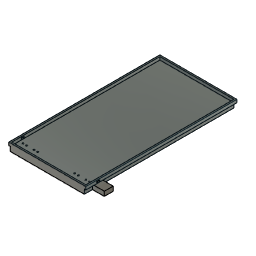
DespotovIdealisticniStoPreKampa v7 (Autodesk Fusion 360 design; units mm, degrees)
Autodesk Fusion 360 part; units mm, degrees
sketch "Sketch1" plane through (0, 0, 0) normal (0, 0, 1) x (1, 0, 0)
  line L0 (0, 0) -> (50, 0)
  line L1 (50, 0) -> (50, 100)
  line L2 (50, 100) -> (0, 100)
  line L3 (0, 100) -> (0, 0)
  constraint horizontal L0
  constraint vertical L1
  constraint horizontal L2
  constraint vertical L3
  constraint coincident L0.start L3.end
extrude "Extrude1" add sketch "Sketch1" along normal blind 3 makes body 1
sketch "Sketch2" plane through (0, 0, 3) normal (0, 0, 1) x (-1, 0, 0)
  line L0 (0, -100) -> (0, 0)
  line L1 (0, 0) -> (-50, 0)
  line L2 (-50, 0) -> (-50, -100)
  line L3 (-50, -100) -> (0, -100)
  line L4 (-50, 0) -> (0, 0)
  line L5 (0, 0) -> (0, 1)
  line L6 (0, 1) -> (-50, 1)
  line L7 (-50, 1) -> (-50, 0)
  line L8 (0, 1) -> (1, 1)
  line L9 (1, 1) -> (1, -100)
  line L10 (1, -100) -> (0, -100)
  line L11 (0, -100) -> (0, 1)
  line L12 (-50, 1) -> (-51, 1)
  line L13 (-51, 1) -> (-51, -100)
  line L14 (-51, -100) -> (-50, -100)
  line L15 (-50, -100) -> (-50, 1)
  line L16 (-51, -100) -> (1, -100)
  line L17 (1, -100) -> (1, -101)
  line L18 (1, -101) -> (-51, -101)
  line L19 (-51, -101) -> (-51, -100)
  constraint horizontal L4
  constraint vertical L5
  constraint horizontal L6
  constraint vertical L7
  constraint coincident L1.end L2.start
  constraint horizontal L8
  constraint vertical L9
  constraint horizontal L10
  constraint vertical L11
  constraint horizontal L12
  constraint vertical L13
  constraint horizontal L14
  constraint vertical L15
  constraint horizontal L16
  constraint vertical L17
  constraint horizontal L18
  constraint vertical L19
extrude "Extrude2" add sketch "Sketch2" along normal blind 2 separate body contours L3 L10 L14 L16 L17 L18 L19 | L0 L5 L8 L9 L10 L11 L16 | L1 L4 L5 L6 L7 L11 L15 | L2 L7 L12 L13 L14 L15 L16 makes body 2
sketch "Sketch3" plane through (0, 0, 3) normal (0, 0, 1) x (-1, 0, 0)
  line L0 (0, -100) -> (0, 0)
  line L1 (0, 0) -> (-50, 0)
  line L2 (-50, 0) -> (-50, -100)
  line L3 (-50, -100) -> (0, -100)
  circle A0 centre (-25, -0.9724) radius 1.0004
extrude "Extrude3" cut sketch "Sketch3" against normal blind 6 contours L1 A0 picked at (-24.8419, -0.7217) bodies 1
sketch "Sketch4" plane through (0, 0, 3) normal (0, 0, 1) x (-1, 0, 0)
  arc A0 (-25.2348, 0) -> (-24.7652, 0) centre (-25, -0.9724) ccw
  line L0 (-25.2348, 0) -> (-50, 0)
  line L1 (-50, 0) -> (-50, -100)
  line L2 (-50, -100) -> (0, -100)
  line L3 (0, -100) -> (0, 0)
  line L4 (0, 0) -> (-24.7652, 0)
  line L5 (-50, 0) -> (0, 0)
  line L6 (0, 0) -> (0, -2)
  line L7 (0, -2) -> (-50, -2)
  line L8 (-50, -2) -> (-50, 0)
  constraint horizontal L5
  constraint vertical L6
  constraint horizontal L7
  constraint vertical L8
  constraint coincident L3 L6.end
  constraint coincident L0.end L1.start
extrude "Extrude4" cut sketch "Sketch4" against normal blind 5 contours A0 L0 L1 L3 L4 L5 L6 L7 L8 bodies 1
sketch "Sketch5" plane through (0, 2, 0) normal (0, -1, 0) x (1, 0, 0)
  line L0 (0, 0) -> (50, 0)
  line L1 (50, 0) -> (50, 3)
  line L2 (50, 3) -> (0, 3)
  line L3 (0, 3) -> (0, 0)
  line L4 (23, 0) -> (0, 3)
  line L5 (0, 0) -> (0, 3)
  line L6 (0, 0) -> (23, 0)
  line L7 (27, 0) -> (50, 3)
  line L8 (50, 0) -> (50, 3)
  line L9 (50, 0) -> (27, 0)
  constraint coincident L0 L4.start
  constraint coincident L2.end L3.start
  constraint coincident L0.start L3.end
  constraint perpendicular L5 L6
  constraint coincident L0 L7.start
  constraint coincident L1.end L2.start
  constraint coincident L0.end L1.start
extrude "Extrude5" add sketch "Sketch5" along normal blind 2 contours L0 L1 L7 L8 L9 bodies 1 2
sketch "Sketch6" plane through (0, 2, 0) normal (0, -1, 0) x (1, 0, 0)
  line L0 (27, 0) -> (50, 3)
  line L1 (50, 3) -> (0, 3)
  line L2 (0, 3) -> (0, 0)
  line L3 (0, 0) -> (27, 0)
  line L4 (23, 0) -> (0, 3)
  line L5 (0, 0) -> (0, 3)
  line L6 (0, 0) -> (23, 0)
  constraint coincident L3 L4.start
  constraint coincident L1.end L2.start
  constraint coincident L2.end L3.start
  constraint perpendicular L5 L6
extrude "Extrude6" add sketch "Sketch6" along normal blind 2 separate body contours L2 L3 L4 L5 L6 makes body 3
sketch "Sketch7" plane through (0, 0, 0) normal (0, -1, 0) x (1, 0, 0)
  line L0 (0, 0) -> (23, 0)
  line L1 (23, 0) -> (0, 3)
  line L2 (0, 3) -> (0, 0)
  line L3 (0, 3) -> (50, 3)
  line L4 (50, 3) -> (50, 0)
  line L5 (50, 0) -> (0, 0)
  line L6 (0, 0) -> (0, 3)
  constraint horizontal L3
  constraint vertical L4
  constraint horizontal L5
  constraint vertical L6
  constraint coincident L1.end L2.start
extrude "Extrude7" add sketch "Sketch7" along normal blind 1 bodies 3 1
sketch "Sketch8" plane through (51, 0, 0) normal (1, 0, 0) x (0, 1, 0)
  line L0 (-1, 3) -> (101, 3)
  line L1 (101, 3) -> (101, 5)
  line L2 (101, 5) -> (-1, 5)
  line L3 (-1, 5) -> (-1, 3)
sketch "Sketch9" plane through (0, 0, 3) normal (0, 0, 1) x (-1, 0, 0)
  line L0 (0, -2) -> (-50, -2)
  line L1 (-50, -2) -> (-50, -100)
  line L2 (-50, -100) -> (0, -100)
  line L3 (0, -100) -> (0, -2)
  circle A0 centre (-47.5, -5) radius 0.5
  circle A1 centre (-45, -5) radius 0.5
  circle A2 centre (-40, -5) radius 0.5
  circle A3 centre (-37.5, -5) radius 0.5
  circle A4 centre (-2.5, -5) radius 0.5
  circle A5 centre (-5, -5) radius 0.5
  circle A6 centre (-10, -5) radius 0.5
  circle A7 centre (-12.5, -5) radius 0.5
  dimension "d15" = 1
  dimension "d16" = 1
  dimension "d17" = 1
  dimension "d18" = 1
  dimension "d19" = 1
  dimension "d20" = 1
  dimension "d21" = 1
  dimension "d22" = 1
  measures "d15" diameter of A0
  measures "d16" diameter of A1
  measures "d17" diameter of A2
  measures "d18" diameter of A3
  measures "d19" diameter of A4
  measures "d20" diameter of A5
  measures "d21" diameter of A6
  measures "d22" diameter of A7
extrude "Extrude8" cut sketch "Sketch9" against normal blind 5 contours A0 | A1 | A2 | A3 | A4 | A5 | A6 | A7 bodies 3
sketch "Sketch10" plane through (51, 0, 0) normal (1, 0, 0) x (0, 1, 0)
  circle A0 centre (8, 4) radius 0.5
  line L0 (7, 4.5) -> (6.5, 4.5)
  line L1 (6.5, 4.5) -> (6.5, 3.5)
  line L2 (6.5, 3.5) -> (7, 3.5)
  line L3 (7, 3.5) -> (7, 4.5)
  dimension "d25" = 1
  constraint horizontal L0
  constraint vertical L1
  constraint horizontal L2
  constraint vertical L3
  measures "d25" diameter of A0
extrude "Extrude9" cut sketch "Sketch10" against normal blind 500 bodies 3
sketch "Sketch11" plane through (50, 0, 0) normal (1, 0, 0) x (0, 1, 0)
  line L0 (-1, 0) -> (100, 0)
  line L1 (100, 0) -> (100, 3)
  line L2 (100, 3) -> (2, 3)
  line L3 (2, 3) -> (0, 3)
  line L4 (0, 3) -> (-1, 3)
  line L5 (-1, 3) -> (-1, 0)
sketch "Sketch12" plane through (50, 0, 0) normal (1, 0, 0) x (0, 1, 0)
  line L0 (4.5, 3) -> (10.5, 3)
  line L1 (10.5, 3) -> (10.5, 0)
  line L2 (10.5, 0) -> (4.5, 0)
  line L3 (4.5, 0) -> (4.5, 3)
  constraint horizontal L0
  constraint vertical L1
  constraint horizontal L2
  constraint vertical L3
extrude "Extrude10" add sketch "Sketch12" along normal blind 8 separate body makes body 4
sketch "Sketch13" plane through (0, 0, 5) normal (0, 0, 1) x (-1, 0, 0)
  line L0 (0, 0) -> (0, -100)
  line L1 (0, -100) -> (-50, -100)
  line L2 (-50, -100) -> (-50, 0)
  line L3 (-50, 0) -> (0, 0)
  line L4 (1, 1) -> (-51, 1)
  line L5 (-51, 1) -> (-51, -101)
  line L6 (-51, -101) -> (1, -101)
  line L7 (1, -101) -> (1, 1)
